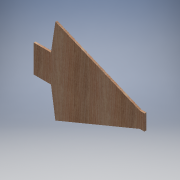
# Autodesk Inventor part: internalSupportBottom1
Saved by Autodesk Inventor 2019 (Build 230136000, 136)
## iProperties
Created: 2019-01-08
Part Number: internalSupportBottom1
Material: Wood (Birch)
Document SubType Name: Modeling
Designer: gaincarlo
Density: 0.55 g/cm^3
Appearance: Birch - Natural Polished
Author: gaincarlo
Autodesk Inventor part; units mm, degrees
ref_plane "YZ Plane" through (0, 0, 0) normal (1, 0, 0) x (0, 1, 0)
ref_plane "XZ Plane" through (0, 0, 0) normal (0, 1, 0) x (-1, 0, 0)
ref_plane "Work Plane1" through (0, 0, 0) normal (0, 0, 1) x (1, 0, 0)
sketch "Sketch1" plane through (0, 0, 0) normal (0, 0, 1) x (1, 0, 0)
  line L0 (-155.0476, 232.0666) -> (-62.9335, 193.9117) construction
  line L1 (177.2752, 94.414) -> (270.7225, 55.7069) construction
  line L2 (177.2752, -94.414) -> (270.7225, -55.7069) construction
  line L3 (-155.0476, -232.0666) -> (-62.9335, -193.9117) construction
  line L4 (-192.4394, 0.4878) -> (-152.8157, 221.8622) construction
  line L5 (-152.8157, -221.8622) -> (-192.4394, -0.4878) construction
  line L6 (302.4733, 35) -> (302.4733, 38) construction
  line L7 (302.4733, -38) -> (302.4733, -35) construction
  line L8 (-254.8213, 5) -> (-254.8213, -5) construction
  line L9 (-272.5267, 75) -> (-179.1025, 75)
  line L10 (-179.1025, 75) -> (-179.1025, -75)
  line L11 (-179.1025, -75) -> (-272.5267, -75)
  line L12 (-272.5267, -75) -> (-272.5267, 75)
  line L13 (327.4733, 53.8478) -> (327.4733, 38) construction
  line L14 (-272.5267, 5) -> (-272.5267, -5) construction
  line L15 (327.4733, 42.5553) -> (302.4733, 42.5553)
  line L16 (302.4733, 42.5553) -> (302.4733, -42.5553)
  line L17 (302.4733, -42.5553) -> (327.4733, -42.5553)
  line L18 (327.4733, -42.5553) -> (327.4733, 42.5553)
  line L19 (-155.0476, 232.0666) -> (302.4733, 42.5553)
  line L20 (-155.0476, -232.0666) -> (302.4733, -42.5553)
  line L21 (-155.0476, 232.0666) -> (-179.1025, 75)
  line L22 (-179.1025, -75) -> (-155.0476, -232.0666)
  point P0 (0, 0)
  point P1 (-151.2693, 230.5016)
  point P2 (-151.2693, -230.5016)
  dimension "d0" = 150
  constraints: 26 end point, 9 point on line, 4 parallel, 2 collinear, 2 horizontal, 2 perpendicular
  measures "d0" distance between parallel lines of L11 L9
extrude "Extrusion1" add sketch "Sketch1" along normal blind 10
body "Solid1"
